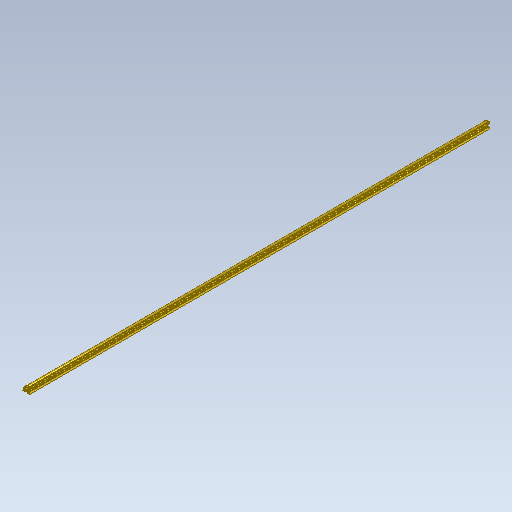
# Autodesk Inventor part: Perfil 30×30 R90 2 rasgos_AST030030R9002
Saved by Autodesk Inventor 2025.2 (Build 292293000, 293)
## iProperties
Created: 2025-04-06
Part Number: Perfil 30×30 R90 2 rasgos_AST030030R9002
Material: Ouro
Document SubType Name: Modeling
Designer: Gustavo Sousa
Density: 19.3 g/cm^3
Appearance: Metal quente 2400F
Author: Gustavo Sousa
Autodesk Inventor part; units mm, degrees
ref_plane "YZ Plane" through (0, 0, 0) normal (1, 0, 0) x (0, 1, 0)
ref_plane "XZ Plane" through (0, 0, 0) normal (0, 1, 0) x (-1, 0, 0)
ref_plane "XY Plane" through (0, 0, 0) normal (0, 0, 1) x (1, 0, 0)
sketch "Esboço1" plane through (0, 0, 0) normal (0, 0, 1) x (1, 0, 0)
  circle A0 centre (0, 0) radius 5 construction
  line L0 (-15, -15) -> (15, -15) construction
  line L1 (-5.4444, -7) -> (5.4444, -7) construction
  line L2 (-4.1, -15) -> (4.1, -15) construction
  line L3 (-4.1, -15) -> (-4.6, -15) construction
  line L4 (-4.6, -15) -> (-4.6, -14.5)
  line L5 (-4.6, -14.5) -> (-4.1, -14.5)
  line L6 (-4.1, -14.5) -> (-4.1, -15) construction
  line L7 (-4.1, -15) -> (-4.1, -12.8) construction
  line L8 (-4.1, -12.8) -> (-7.9, -12.8) construction
  line L9 (-4.1, -12.8) -> (-4.1, -14.5)
  line L10 (-15, -15) -> (-15, 15) construction
  line L11 (-15, 15) -> (15, 15) construction
  line L12 (15, 15) -> (15, -15) construction
  line L13 (4.1, -15) -> (4.6, -15) construction
  line L14 (4.6, -15) -> (4.6, -14.5)
  line L15 (4.6, -14.5) -> (4.1, -14.5)
  line L16 (4.1, -14.5) -> (4.1, -15) construction
  arc A1 (14.5, -15) -> (15, -14.5) centre (14.5, -14.5) ccw
  line L17 (4.6, -15) -> (14.5, -15)
  line L18 (4.1, -12.8) -> (4.1, -15) construction
  line L19 (4.1, -12.8) -> (7.9, -12.8) construction
  line L20 (4.1, -12.8) -> (4.1, -14.5)
  line L21 (0, 0) -> (15, -15)
  line L22 (5.4444, -7) -> (7.9, -9.4556) construction
  line L23 (7.9, -12.8) -> (7.9, -9.4556) construction
  circle A2 centre (11.5, -11.5) radius 2.5
  line L24 (-7.9, -9.4556) -> (-7.9, -12.8) construction
  line L25 (0, 0) -> (-15, -15) construction
  line L26 (-7.9, -9.4556) -> (-5.4444, -7) construction
  arc A3 (-15, -14.5) -> (-14.5, -15) centre (-14.5, -14.5) ccw
  line L27 (-14.5, -15) -> (-4.6, -15)
  line L28 (0, 0) -> (-15, 15) construction
  line L29 (-10.1, -8.5444) -> (-6.4546, -4.899) construction
  line L30 (-10.1, -8.5444) -> (-10.1, -13.65) construction
  line L31 (-13.75, -13.65) -> (-10.1, -13.65) construction
  line L32 (-13.75, -13.65) -> (-13.75, -13.15) construction
  arc A4 (-13.75, -13.15) -> (-13.25, -13.65) centre (-13.25, -13.15) ccw
  arc A5 (-10.6, -13.65) -> (-10.1, -13.15) centre (-10.6, -13.15) ccw
  arc A6 (-7.9, -12.3) -> (-7.4, -12.8) centre (-7.4, -12.3) ccw
  arc A7 (-7.7536, -9.3092) -> (-7.9, -9.6627) centre (-7.4, -9.6627) ccw
  arc A8 (-5.2373, -7) -> (-5.5908, -7.1464) centre (-5.2373, -7.5) ccw
  arc A9 (5.5908, -7.1464) -> (5.2373, -7) centre (5.2373, -7.5) ccw
  arc A10 (7.9, -9.6627) -> (7.7536, -9.3092) centre (7.4, -9.6627) ccw
  arc A11 (7.4, -12.8) -> (7.9, -12.3) centre (7.4, -12.3) ccw
  line L33 (-7.4, -12.8) -> (-4.1, -12.8)
  line L34 (-7.9, -12.3) -> (-7.9, -9.6627)
  line L35 (-7.7536, -9.3092) -> (-5.5908, -7.1464)
  line L36 (-5.2373, -7) -> (5.2373, -7)
  line L37 (5.5908, -7.1464) -> (7.7536, -9.3092)
  line L38 (7.9, -9.6627) -> (7.9, -12.3)
  line L39 (7.4, -12.8) -> (4.1, -12.8)
  arc A12 (-9.9536, -8.3979) -> (-10.1, -8.7515) centre (-9.6, -8.7515) ccw
  line L40 (2.6476, -6) -> (6, -6) construction
  line L41 (6, -6) -> (6, -2.6476) construction
  line L42 (6, -2.6476) -> (0, 0) construction
  line L43 (2.6476, -6) -> (0, 0) construction
  line L44 (6, -2.6476) -> (4.5744, -2.0186) construction
  line L45 (2.6476, -6) -> (2.0186, -4.5744) construction
  arc A13 (2.5161, -5.7019) -> (2.9735, -6) centre (2.9735, -5.5) ccw
  arc A14 (5.5, -6) -> (6, -5.5) centre (5.5, -5.5) ccw construction
  arc A15 (2.2112, -5.011) -> (1.5943, -4.739) centre (1.7538, -5.2129) ccw
  arc A16 (-3.5355, 3.5355) -> (1.5943, -4.739) centre (0, 0) ccw
  line L46 (2.2112, -5.011) -> (2.5161, -5.7019)
  line L47 (2.9735, -6) -> (5.5, -6)
  arc A17 (5.5, -6) -> (5.8536, -5.8536) centre (5.5, -5.5) ccw
  line L48 (-10.6, -13.65) -> (-13.25, -13.65)
  line L49 (-10.1, -13.15) -> (-10.1, -8.7515)
  circle A18 centre (0, 0) radius 7 construction
  arc A19 (-4.9497, 4.9497) -> (-7, 0) centre (0, 0) ccw construction
  arc A20 (-7, 0) -> (-5.6695, -4.1057) centre (0, 0) ccw
  line L50 (-15, 0) -> (0, 15) construction
  arc A21 (14.5, 15) -> (-15, -14.5) centre (14.5, -14.5) ccw construction
  line L51 (0, 0) -> (15, 15) construction
  arc A22 (15, 14.5) -> (14.5, 15) centre (14.5, 14.5) ccw construction
  arc A23 (-7.9672, 2.6788) -> (-13.75, -13.15) centre (14.5, -14.5) ccw construction
  arc A24 (-4.9497, 4.9497) -> (-7, 0) centre (0, 0) ccw construction
  line L52 (-6.4672, 2.6788) -> (-7.9672, 2.6788) construction
  arc A25 (-6.7936, 1.6874) -> (-8.2103, 2.356) centre (-7.5689, 1.8799) ccw
  arc A26 (-6.4672, 2.6788) -> (-7, 0) centre (0, 0) ccw construction
  arc A27 (-8.2103, 2.356) -> (-13.75, -13.15) centre (14.5, -14.5) ccw
  arc A28 (-6.7936, 1.6874) -> (-7, 0) centre (0, 0) ccw
  arc A29 (-6.3597, 6.3597) -> (-15, -14.5) centre (14.5, -14.5) ccw
  line L53 (-6.3597, 6.3597) -> (0, 0)
  line L54 (-9.9536, -8.3979) -> (-6.4546, -4.899) construction
  line L55 (-6.6011, -5.0454) -> (-9.9536, -8.3979)
  line L56 (0, 0) -> (-5, 0) construction
  line L57 (-5, 0) -> (-5, -4.899) construction
  line L58 (-6.4546, -4.899) -> (-5, -4.899) construction
  arc A30 (-6.0745, -4.899) -> (-5.6695, -4.1057) centre (-6.0745, -4.399) ccw
  arc A31 (-6.2475, -4.899) -> (-6.6011, -5.0454) centre (-6.2475, -5.399) ccw
  line L59 (-6.2475, -4.899) -> (-6.0745, -4.899)
  point P0 (0, -15)
  point P1 (0, -7)
  point P2 (0, -15)
  point P3 (-4.1, -13.65)
  point P4 (14.8536, -14.8536)
  point P5 (13.2678, -13.2678)
  point P6 (9.7322, -9.7322)
  point P7 (5.8536, -5.8536)
  point P8 (-3.5355, 3.5355)
  point P9 (-5.6695, -4.1057)
  dimension "d0" = 10
  dimension "d1" = 30
  dimension "d2" = 15
  dimension "d3" = 8
  dimension "d4" = 8.2
  dimension "quadrado" = 0.5
  dimension "espessura" = 2.2
  dimension "arco" = 0.5
  dimension "d10" = 11.5
  dimension "d11" = 5
  dimension "d12" = 1.1
  dimension "d13" = 1.1
  dimension "d14" = 1.1
  dimension "d15" = 2.2
  dimension "d16" = 1.25
  dimension "d19" = 1
  dimension "d20" = 42.379
  dimension "d25" = 2
  constraints: 122 end point, 73 point on circle, 46 tangent, 39 point on line, 32 centre point, 23 equal radius, 15 collinear, 13 horizontal, 10 equal length, 8 vertical, 7 coincident, 7 parallel, 6 midpoint, 3 horizontal alignment, 3 perpendicular, 2 concentric, 2 vertical alignment, 5 other
  measures "d0" diameter of A0
  measures "d1" distance of L0.start L0.end
  measures "d2" distance of point (0, 0) point (0, -15)
  measures "d3" distance between parallel lines of L0 L1
  measures "d4" distance of L2.start L2.end
  measures "quadrado" distance of L5.end L2.start
  measures "espessura" distance between parallel lines of L0 L8
  measures "arco" radius of A1
  measures "d10" horizontal distance of point (0, 0) A2.centre
  measures "d11" diameter of A2
  measures "d12" distance edge to line of A2 L23
  measures "d13" distance between parallel lines of L21 L22
  measures "d14" distance between parallel lines of L25 L29
  measures "d15" distance between parallel lines of L24 L30
  measures "d16" distance between parallel lines of L10 L32
  measures "d19" distance between parallel lines of L1 L40
  measures "d20" angle of L43 L42
  measures "d25" radial gap between concentric circles of A0 A20
extrude "Extrusão1" add sketch "Esboço1" along normal mid plane 2000 contours L27 A3 A29 L53 A16 A15 L46 A13 L47 A17 L21 A2 A1 L17 L14 L15 L20 L39 A11 L38 A10 L37 A9 L36 A8 L35 A7 L34 A6 L33 L9 L5 L4
mirror "Espelhar1" about plane through (-3.5355, 3.5355, 0) normal (0.7071068, 0.7071068, 0) of "Extrusão1"
equation "\"d12\" = 0.5 * espessura"
equation "\"d13\" = 0.5 * espessura"
equation "\"d15\" = espessura"
